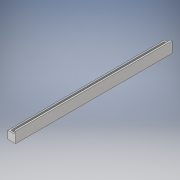
# Autodesk Inventor part: calha
Saved by Autodesk Inventor 2019.4 (Build 234330000, 330)
## iProperties
Created: 2020-04-10
Part Number: calha
Material: Genérico
Document SubType Name: Modeling
Designer: lucas
Density: 1 g/cm^3
Appearance: Padrão
Author: lucas
Autodesk Inventor part; units mm, degrees
ref_plane "YZ Plane" through (0, 0, 0) normal (1, 0, 0) x (0, 1, 0)
ref_plane "XZ Plane" through (0, 0, 0) normal (0, 1, 0) x (-1, 0, 0)
ref_plane "XY Plane" through (0, 0, 0) normal (0, 0, 1) x (1, 0, 0)
sketch "Esboço1" plane through (0, 0, 0) normal (0, 0, 1) x (1, 0, 0)
  line L0 (0, 0) -> (50, 0)
  line L1 (50, 0) -> (50, 70)
  line L2 (50, 70) -> (40, 70)
  line L3 (40, 70) -> (40, 10)
  line L4 (40, 10) -> (10, 10)
  line L5 (10, 10) -> (10, 50)
  line L6 (10, 50) -> (0, 50)
  line L7 (0, 50) -> (0, 0)
  dimension "d0" = 10
  dimension "d1" = 10
  dimension "d2" = 10
  dimension "d3" = 50
  dimension "d4" = 50
  dimension "d5" = 70
  constraints: 16 end point, 7 perpendicular, 1 horizontal
  measures "d0" distance between parallel lines of L5 L7
  measures "d1" distance between parallel lines of L0 L4
  measures "d2" distance between parallel lines of L1 L3
  measures "d3" distance between parallel lines of L1 L7
  measures "d4" distance between parallel lines of L0 L6
  measures "d5" distance between parallel lines of L0 L2
extrude "Extrusão1" add sketch "Esboço1" along normal blind 1010
sketch "Esboço2" plane through (0, 0, 1010) normal (0, 0, 1) x (1, 0, 0)
  line L0 (0, 0) -> (50, 0) projected
  line L1 (0, 0) -> (50, 0)
  line L2 (50, 0) -> (50, 50)
  line L3 (50, 50) -> (0, 50)
  line L4 (10, 10) -> (10, 50) projected
  line L5 (0, 50) -> (0, 0) projected
  line L6 (0, 50) -> (0, 0)
  constraints: 8 end point, 2 perpendicular, 1 collinear, 1 horizontal
extrude "Extrusão2" add sketch "Esboço2" against normal blind 10
sketch "Esboço3" plane through (0, 0, 0) normal (0, 0, -1) x (-1, 0, 0)
  line L0 (0, 0) -> (-50, 0) projected
  line L1 (-40, 50) -> (0, 50) projected
  line L2 (-50, 0) -> (0, 0)
  line L3 (0, 0) -> (0, 50)
  line L4 (0, 50) -> (-50, 50)
  line L5 (-50, 50) -> (-50, 0)
  constraints: 8 end point, 2 parallel, 1 horizontal, 1 perpendicular
extrude "Extrusão3" add sketch "Esboço3" against normal blind 10
